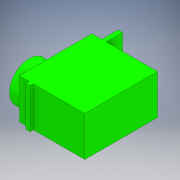
# Autodesk Inventor part: Servo
Saved by Autodesk Inventor 2018 (Build 220112000, 112)
## iProperties
Created: 2018-01-06
Part Number: Servo
Material: Generic
Document SubType Name: Modeling
Designer: suchanek
Density: 1 g/cm^3
Appearance: Default
Mass: 5.85125 g
Surface Area: 21.9278 cm^2
Volume: 5.85125 cm^3
Author: suchanek
Autodesk Inventor part; units mm, degrees
ref_plane "YZ Plane" through (0, 0, 0) normal (1, 0, 0) x (0, 1, 0)
ref_plane "XZ Plane" through (0, 0, 0) normal (0, 1, 0) x (-1, 0, 0)
ref_plane "XY Plane" through (0, 0, 0) normal (0, 0, 1) x (1, 0, 0)
sketch "Sketch1" plane through (0, 0, 0) normal (0, 0, 1) x (1, 0, 0)
  line L0 (0, 0) -> (20, 0)
  line L1 (20, 0) -> (20, 22.2)
  line L2 (20, 22.2) -> (0, 22.2)
  line L3 (0, 22.2) -> (0, 0)
  dimension "d0" = 20
  dimension "d1" = 22.2
  constraints: 8 end point, 2 parallel, 1 horizontal, 1 perpendicular
  measures "d0" distance of L2.end L1.end
  measures "d1" distance of L1.end L0.end
extrude "Extrusion1" add sketch "Sketch1" along normal mid plane 12.2
sketch "Sketch2" plane through (0, 0, 6.1) normal (-1, 0, 0) x (0, 0, 1)
  circle A0 centre (-6, 6) radius 6
  line L0 (0, 0) -> (-12.2, 0) projected
  line L1 (0, 22.2) -> (0, 0) projected
  point P0 (-6.1, 0)
  dimension "d4" = 6
  dimension "d5" = 6
  dimension "d6" = 12
  constraints: 1 centre point
  measures "d4" distance from line of A0.centre L0
  measures "d5" distance from line of L1 A0.centre
  measures "d6" diameter of A0
extrude "Extrusion2" add sketch "Sketch2" along normal blind 3 contours A0
sketch "Sketch3" plane through (0, 22.2, 6.1) normal (0, 1, 0) x (1, 0, 0)
  line L0 (0, 0) -> (20, 0) projected
  line L1 (3, 12.2) -> (4.3, 12.2)
  line L2 (4.3, 12.2) -> (4.3, 0)
  line L3 (4.3, 0) -> (3, 0)
  line L4 (3, 0) -> (3, 12.2)
  line L5 (0, 12.2) -> (0, 0) projected
  point P0 (0, 6.1)
  dimension "d9" = 3
  dimension "d10" = 1.3
  dimension "d11" = 12.2
  constraints: 8 end point, 2 parallel, 1 horizontal, 1 perpendicular, 1 point on line
  measures "d9" distance between parallel lines of L4 L5
  measures "d10" distance between parallel lines of L2 L4
  measures "d11" distance between parallel lines of L0 L1
extrude "Extrusion3" add sketch "Sketch3" along normal blind 5 and the other way blind 27.2
sketch "Sketch5" plane through (4.3, -5, 6.1) normal (1, 0, 0) x (0, 0, -1)
  line L0 (0, 0) -> (12.2, 0)
  line L1 (12.2, 0) -> (12.2, 4)
  line L2 (12.2, 4) -> (0, 4)
  line L3 (0, 4) -> (0, 0)
  line L4 (0, 5) -> (0, 0) projected
  line L5 (12.2, 5) -> (12.2, 0) projected
  line L6 (12.2, 0) -> (0, 0) projected
  line L7 (12.2, 5) -> (0, 5) projected
  point P0 (6.1, 5)
  dimension "d24" = 1
  constraints: 8 end point, 3 collinear, 2 parallel, 1 horizontal, 1 perpendicular
  measures "d24" distance between parallel lines of L7 L2
extrude "Extrusion5" cut sketch "Sketch5" against normal blind 2 contours L3 L2 L1 L0
body "Solid1"
